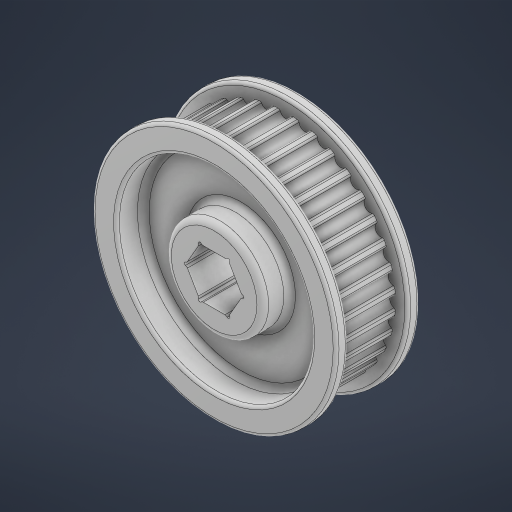
# Autodesk Inventor part: 5 mm HTD Pulley
Saved by Autodesk Inventor 2023.1 (Build 271208000, 208)
## iProperties
Created: 2022-03-07
Part Number: 5 mm HTD Pulley
Material: Phenolic Resin
Document SubType Name: Modeling
Designer: Byron Robotics
Mass: 46.2989 g
Surface Area: 159.635 cm^2
Volume: 33.5499 cm^3
Density: 1.38 g/cm^3
Appearance: Smooth - Light Gray
Description: Parametric 5 mm HTD Pulley for 3D Printing
Author: Byron Robotics
Revision Number: A
Autodesk Inventor part; units mm, degrees
ref_plane "YZ Plane" through (0, 0, 0) normal (1, 0, 0) x (0, 1, 0)
ref_plane "XZ Plane" through (0, 0, 0) normal (0, 1, 0) x (-1, 0, 0)
sketch "Pitch Diameter" plane through (0, 0, 0) normal (0, 0, 1) x (1, 0, 0)
  circle A0 centre (0, 0) radius 28.6479
  dimension "d13" = 57.2958
  constraints: 1 centre point, 1 coincident
  measures "d13" diameter of A0
extrude "Extrusion1" add sketch "Pitch Diameter" along normal blind 15.5
sketch "TeethCut" plane through (0, 0, 0) normal (0, 0, 1) x (1, 0, 0)
  circle A0 centre (0, 28.6479) radius 1.525
  line L0 (0, 30.1729) -> (0, 29.1829) construction
  line L1 (0, 30.1729) -> (5.4407, 30.1729) construction
  line L2 (0, 0) -> (0, 29.1829) construction
  circle A1 centre (0, 0) radius 28.6479 construction
  circle A2 centre (0, 0) radius 30.9229 construction
  line L3 (0, 27.1229) -> (0, 30.9229) construction
  circle A3 centre (-4.9747, 28.2127) radius 1.525
  circle A4 centre (-9.7982, 26.9202) radius 1.525
  circle A5 centre (-14.3239, 24.8098) radius 1.525
  circle A6 centre (-18.4145, 21.9456) radius 1.525
  circle A7 centre (-21.9456, 18.4145) radius 1.525
  circle A8 centre (-24.8098, 14.3239) radius 1.525
  circle A9 centre (-26.9202, 9.7982) radius 1.525
  circle A10 centre (-28.2127, 4.9747) radius 1.525
  circle A11 centre (-28.6479, 0) radius 1.525
  circle A12 centre (-28.2127, -4.9747) radius 1.525
  circle A13 centre (-26.9202, -9.7982) radius 1.525
  circle A14 centre (0, 0) radius 29.1829 construction
  circle A15 centre (-24.8098, -14.3239) radius 1.525
  circle A16 centre (-21.9456, -18.4145) radius 1.525
  circle A17 centre (-18.4145, -21.9456) radius 1.525
  circle A18 centre (-14.3239, -24.8098) radius 1.525
  circle A19 centre (-9.7982, -26.9202) radius 1.525
  circle A20 centre (-4.9747, -28.2127) radius 1.525
  circle A21 centre (0, -28.6479) radius 1.525
  circle A22 centre (4.9747, -28.2127) radius 1.525
  circle A23 centre (9.7982, -26.9202) radius 1.525
  circle A24 centre (14.3239, -24.8098) radius 1.525
  circle A25 centre (18.4145, -21.9456) radius 1.525
  circle A26 centre (21.9456, -18.4145) radius 1.525
  circle A27 centre (24.8098, -14.3239) radius 1.525
  circle A28 centre (26.9202, -9.7982) radius 1.525
  circle A29 centre (28.2127, -4.9747) radius 1.525
  circle A30 centre (28.6479, 0) radius 1.525
  circle A31 centre (28.2127, 4.9747) radius 1.525
  circle A32 centre (26.9202, 9.7982) radius 1.525
  circle A33 centre (24.8098, 14.3239) radius 1.525
  circle A34 centre (21.9456, 18.4145) radius 1.525
  circle A35 centre (18.4145, 21.9456) radius 1.525
  circle A36 centre (14.3239, 24.8098) radius 1.525
  circle A37 centre (9.7982, 26.9202) radius 1.525
  circle A38 centre (4.9747, 28.2127) radius 1.525
  point P0 (-5.2395, 29.7145)
  point P1 (-4.7098, 26.7108)
  point P2 (-10.3197, 28.3532)
  point P3 (-9.2766, 25.4872)
  point P4 (-15.0864, 26.1305)
  point P5 (-13.5614, 23.4891)
  point P6 (-19.3948, 23.1138)
  point P7 (-17.4343, 20.7773)
  point P8 (-23.1138, 19.3948)
  point P9 (-20.7773, 17.4343)
  point P10 (-26.1305, 15.0864)
  point P11 (-23.4891, 13.5614)
  point P12 (-28.3532, 10.3197)
  point P13 (-25.4872, 9.2766)
  point P14 (-29.7145, 5.2395)
  point P15 (-26.7108, 4.7098)
  point P16 (-30.1729, 0)
  point P17 (-27.1229, 0)
  point P18 (-29.7145, -5.2395)
  point P19 (-26.7108, -4.7098)
  point P20 (-28.3532, -10.3197)
  point P21 (-25.4872, -9.2766)
  point P22 (-26.1305, -15.0864)
  point P23 (-23.4891, -13.5614)
  point P24 (-23.1138, -19.3948)
  point P25 (-20.7773, -17.4343)
  point P26 (-19.3948, -23.1138)
  point P27 (-17.4343, -20.7773)
  point P28 (-15.0864, -26.1305)
  point P29 (-13.5614, -23.4891)
  point P30 (-10.3197, -28.3532)
  point P31 (-9.2766, -25.4872)
  point P32 (-5.2395, -29.7145)
  point P33 (-4.7098, -26.7108)
  point P34 (0, -30.1729)
  point P35 (0, -27.1229)
  point P36 (5.2395, -29.7145)
  point P37 (4.7098, -26.7108)
  point P38 (10.3197, -28.3532)
  point P39 (9.2766, -25.4872)
  point P40 (15.0864, -26.1305)
  point P41 (13.5614, -23.4891)
  point P42 (19.3948, -23.1138)
  point P43 (17.4343, -20.7773)
  point P44 (23.1138, -19.3948)
  point P45 (20.7773, -17.4343)
  point P46 (26.1305, -15.0864)
  point P47 (23.4891, -13.5614)
  point P48 (28.3532, -10.3197)
  point P49 (25.4872, -9.2766)
  point P50 (29.7145, -5.2395)
  point P51 (26.7108, -4.7098)
  point P52 (30.1729, 0)
  point P53 (27.1229, 0)
  point P54 (29.7145, 5.2395)
  point P55 (26.7108, 4.7098)
  point P56 (28.3532, 10.3197)
  point P57 (25.4872, 9.2766)
  point P58 (26.1305, 15.0864)
  point P59 (23.4891, 13.5614)
  point P60 (23.1138, 19.3948)
  point P61 (20.7773, 17.4343)
  point P62 (19.3948, 23.1138)
  point P63 (17.4343, 20.7773)
  point P64 (15.0864, 26.1305)
  point P65 (13.5614, 23.4891)
  point P66 (10.3197, 28.3532)
  point P67 (9.2766, 25.4872)
  point P68 (5.2395, 29.7145)
  point P69 (4.7098, 26.7108)
  dimension "d7" = 57.2958
  dimension "d2" = 3.05
  dimension "TipToBackBeltHeight" = 3.8
  dimension "d10" = 360
  dimension "d12" = 1.74
  constraints: 72 point on circle, 36 centre point, 8 end point, 4 coincident, 3 point on line, 3 vertical alignment, 1 collinear, 1 horizontal, 1 perpendicular, 1 tangent, 151 other
  measures "d2" diameter of A0
  measures "TipToBackBeltHeight" distance of L3.start L3.end
  measures "d12" distance of L0.end L3.end
extrude "Extrusion3" cut sketch "TeethCut" along normal through all contours A0
fillet "Fillet1" radius 0.5 2 edges at (1.5245, 28.6073, 7.75) (-1.5245, 28.6073, 7.75)
pattern_circular "Circular Pattern1" count 36 over 360 about axis through (0, 0, 0) along (0, 0, 1) of "Extrusion3", "Fillet1"
ref_plane "Work Plane1" through (0, 0, 7.75) normal (0, 0, 1) x (1, 0, 0)
sketch "Sketch4" plane through (0, 0, 15.5) normal (0, 0, 1) x (1, 0, 0)
  circle A0 centre (0, 0) radius 31.8229
  dimension "d26" = 63.6458
  constraints: 1 centre point, 1 coincident
  measures "d26" diameter of A0
extrude "Extrusion4" add sketch "Sketch4" along normal blind 3.175
mirror "Mirror1" about plane through (0, 0, 7.75) normal (0, 0, 1) of "Extrusion4"
fillet "Fillet2" radius 0.762 4 edges at (-31.8229, 0, 18.675) (-31.8229, 0, 15.5) (-31.8229, 0, 0) (-31.8229, 0, -3.175)
sketch "Sketch5" plane through (0, 0, 18.675) normal (0, 0, 1) x (1, 0, 0)
  line L0 (3.6882, 6.3881) -> (7.3763, 0)
  line L1 (7.3763, 0) -> (3.6882, -6.3881)
  line L2 (3.6882, -6.3881) -> (-3.6882, -6.3881)
  line L3 (-3.6882, -6.3881) -> (-7.3763, 0)
  line L4 (-7.3763, 0) -> (-3.6882, 6.3881)
  line L5 (-3.6882, 6.3881) -> (3.6882, 6.3881)
  circle A0 centre (-3.6882, 6.3881) radius 0.381
  circle A1 centre (3.6882, 6.3881) radius 0.381
  circle A2 centre (7.3763, 0) radius 0.381
  circle A3 centre (3.6882, -6.3881) radius 0.381
  circle A4 centre (-3.6882, -6.3881) radius 0.381
  circle A5 centre (-7.3763, 0) radius 0.381
  point P0 (0, 0)
  point P1 (0, 0)
  point P2 (-7.1858, -0.33)
  point P3 (-3.8787, -6.0581)
  point P4 (-3.3072, -6.3881)
  point P5 (3.3072, -6.3881)
  point P6 (3.8787, -6.0581)
  point P7 (7.1858, -0.33)
  point P8 (7.1858, 0.33)
  point P9 (3.8787, 6.0581)
  point P10 (3.3072, 6.3881)
  point P11 (-3.3072, 6.3881)
  point P12 (-3.8787, 6.0581)
  point P13 (-7.1858, 0.33)
  dimension "d30" = 12.7762
  dimension "d31" = 0.762
  constraints: 12 end point, 7 coincident, 6 centre point, 5 equal radius, 1 horizontal, 13 other
  measures "d30" distance between parallel lines of L2 L5
  measures "d31" diameter of A0
extrude "Extrusion5" cut sketch "Sketch5" against normal through all
fillet "Fillet3" radius 0.762 12 edges at (3.3072, 6.3881, 7.75) (3.8787, 6.0581, 7.75) (7.1858, 0.33, 7.75) (7.1858, -0.33, 7.75) (3.8787, -6.0581, 7.75) (3.3072, -6.3881, 7.75) (-3.3072, -6.3881, 7.75) (-3.8787, -6.0581, 7.75) (-7.1858, -0.33, 7.75) (-7.1858, 0.33, 7.75) (-3.3072, 6.3881, 7.75) (-3.8787, 6.0581, 7.75)
sketch "Sketch6" plane through (0, 0, 18.675) normal (0, 0, 1) x (1, 0, 0)
  circle A0 centre (0, 0) radius 25.4729
  circle A1 centre (0, 0) radius 12.7
  dimension "d35" = 25.4
  dimension "d36" = 50.9458
  constraints: 2 centre point, 2 coincident
  measures "d35" diameter of A1
  measures "d36" diameter of A0
extrude "Extrusion6" cut sketch "Sketch6" against normal blind 7
mirror "Mirror2" about plane through (0, 0, 7.75) normal (0, 0, 1) of "Extrusion6"
fillet "Fillet4" radius 0.762 2 edges at (-25.4729, 0, -3.175) (-25.4729, 0, 18.675)
fillet "Fillet5" radius 1.524 2 edges at (-12.7, 0, 18.675) (-12.7, 0, -3.175)
fillet "Fillet6" radius 1.524 4 edges at (-25.4729, 0, 3.825) (-12.7, 0, 3.825) (-12.7, 0, 11.675) (-25.4729, 0, 11.675)
ref_plane "Work Plane2" through (0, 0, 7.75) normal (0, 0, 1) x (1, 0, 0)
equation "\"d13\" = PitchDiameter"
equation "\"d7\" = PitchDiameter"
equation "\"PitchDiameter\" = 57.29578"
body "Solid1"
